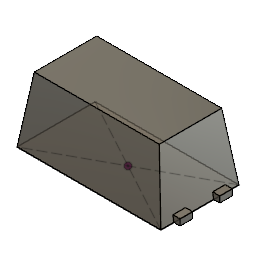
4-Mini-Flat (Autodesk Fusion 360 design; units mm, degrees)
Autodesk Fusion 360 part; units mm, degrees
sketch "Sketch1" plane through (0, 0, 0) normal (0, 1, 0) x (1, 0, 0)
  line L0 (2.3, 1.25) -> (-2.3, 1.25)
  line L1 (-2.3, 1.25) -> (-2.3, -1.25)
  line L2 (-2.3, -1.25) -> (2.3, -1.25)
  line L3 (2.3, -1.25) -> (2.3, 1.25)
  line L4 (2.3, 1.25) -> (-2.3, -1.25) construction
  line L5 (-2.3, 1.25) -> (2.3, -1.25) construction
  dimension "d1" = 4.6
  dimension "d2" = 2.5
  constraint perpendicular L0 L1
  constraint parallel L0 L2
  constraint parallel L1 L3
  constraint horizontal L0
  constraint coincident L4 origin
  constraint coincident L5 origin
  measures "d1" distance of L1.end L2.end
  measures "d2" distance of L0.end L1.end
ref_plane "WorkPlane1" through (0, 2.1, 0) normal (0, 1, 0) x (0, 0, 1)
sketch "Sketch2" plane through (0, 2.1, 0) normal (0, 1, 0) x (1, 0, 0)
  line L0 (2, 1) -> (-2, 1)
  line L1 (-2, 1) -> (-2, -1)
  line L2 (-2, -1) -> (2, -1)
  line L3 (2, -1) -> (2, 1)
  line L4 (2, 1) -> (-2, -1) construction
  line L5 (-2, 1) -> (2, -1) construction
  dimension "d4" = 4
  dimension "d5" = 2
  constraint perpendicular L0 L1
  constraint parallel L0 L2
  constraint parallel L1 L3
  constraint horizontal L0
  constraint coincident L4 origin
  constraint coincident L5 origin
  measures "d4" distance of L1.end L2.end
  measures "d5" distance of L0.end L1.end
loft "Loft1" add profiles "Sketch1", "Sketch2" section 1 section 2
sketch "Sketch3" plane through (0, 0, 0) normal (0, 1, 0) x (1, 0, 0)
  line L0 (-2.3, 1.25) -> (-2.3, -1.25) construction
  line L1 (-2.3, 0) -> (-2.3, 0.635) construction
  line L2 (-2.3, 0) -> (-2.3, -0.635) construction
  line L3 (2.3, -1.25) -> (2.3, 1.25) construction
  line L4 (2.3, 1.25) -> (-2.3, 1.25) construction
  line L5 (2.3, 0) -> (2.3, 0.635) construction
  line L6 (2.3, 0) -> (2.3, -0.635) construction
  line L7 (-2.1, 0.835) -> (-2.5, 0.835)
  line L8 (-2.5, 0.835) -> (-2.5, 0.435)
  line L9 (-2.5, 0.435) -> (-2.1, 0.435)
  line L10 (-2.1, 0.435) -> (-2.1, 0.835)
  line L11 (-2.1, 0.835) -> (-2.5, 0.435) construction
  line L12 (-2.5, 0.835) -> (-2.1, 0.435) construction
  line L13 (-2.1, -0.435) -> (-2.5, -0.435)
  line L14 (-2.5, -0.435) -> (-2.5, -0.835)
  line L15 (-2.5, -0.835) -> (-2.1, -0.835)
  line L16 (-2.1, -0.835) -> (-2.1, -0.435)
  line L17 (-2.1, -0.435) -> (-2.5, -0.835) construction
  line L18 (-2.5, -0.435) -> (-2.1, -0.835) construction
  line L19 (2.5, 0.835) -> (2.1, 0.835)
  line L20 (2.1, 0.835) -> (2.1, 0.435)
  line L21 (2.1, 0.435) -> (2.5, 0.435)
  line L22 (2.5, 0.435) -> (2.5, 0.835)
  line L23 (2.5, 0.835) -> (2.1, 0.435) construction
  line L24 (2.1, 0.835) -> (2.5, 0.435) construction
  line L25 (2.5, -0.435) -> (2.1, -0.435)
  line L26 (2.1, -0.435) -> (2.1, -0.835)
  line L27 (2.1, -0.835) -> (2.5, -0.835)
  line L28 (2.5, -0.835) -> (2.5, -0.435)
  line L29 (2.5, -0.435) -> (2.1, -0.835) construction
  line L30 (2.1, -0.435) -> (2.5, -0.835) construction
  point P0 (-2.3, 0.635)
  point P1 (-2.3, -0.635)
  point P2 (2.3, 0.635)
  point P3 (2.3, -0.635)
  dimension "d6" = 0.635
  dimension "d7" = 0.635
  dimension "d8" = 0.635
  dimension "d9" = 0.635
  dimension "d10" = 0.4
  dimension "d11" = 0.4
  dimension "d12" = 0.4
  dimension "d13" = 0.4
  dimension "d14" = 0.4
  dimension "d15" = 0.4
  dimension "d16" = 0.4
  dimension "d17" = 0.4
  constraint midpoint L0 L1.start
  constraint parallel L0 L1
  constraint parallel L0 L2
  constraint midpoint L3 L5.start
  constraint perpendicular L4 L5
  constraint parallel L3 L6
  constraint perpendicular L7 L8
  constraint parallel L7 L9
  constraint parallel L8 L10
  constraint horizontal L7
  constraint coincident L11 P0
  constraint coincident L12 P0
  constraint coincident P0 L1.end
  constraint perpendicular L13 L14
  constraint parallel L13 L15
  constraint parallel L14 L16
  constraint horizontal L13
  constraint coincident L17 P1
  constraint coincident L18 P1
  constraint coincident P1 L2.end
  constraint perpendicular L19 L20
  constraint parallel L19 L21
  constraint parallel L20 L22
  constraint horizontal L19
  constraint coincident L23 P2
  constraint coincident L24 P2
  constraint coincident P2 L5.end
  constraint perpendicular L25 L26
  constraint parallel L25 L27
  constraint parallel L26 L28
  constraint horizontal L25
  constraint coincident L29 P3
  constraint coincident L30 P3
  constraint coincident P3 L6.end
  measures "d6" distance of L1.start P0
  measures "d7" distance of L1.start P1
  measures "d8" distance of L5.start P2
  measures "d9" distance of L5.start P3
  measures "d10" distance of L8.end L9.end
  measures "d11" distance of L7.end L8.end
  measures "d12" distance of L14.end L15.end
  measures "d13" distance of L13.end L14.end
  measures "d14" distance of L19.end L20.end
  measures "d15" distance of L20.end L21.end
  measures "d16" distance of L26.end L27.end
  measures "d17" distance of L25.end L26.end
extrude "Extrude1" add sketch "Sketch3" along normal blind 0.2
